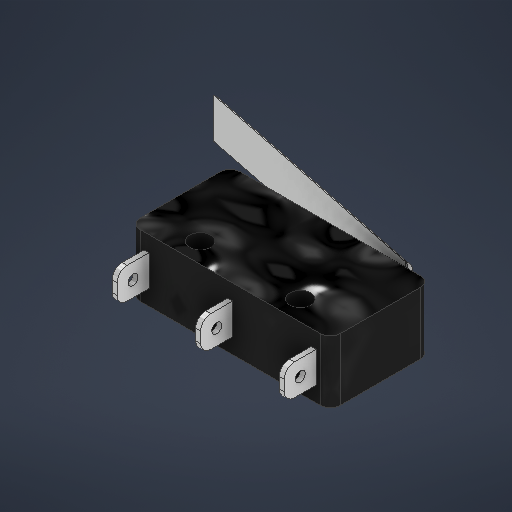
# Autodesk Inventor part: switch
Saved by Autodesk Inventor 2026.1 (Build 301233000, 233)
## iProperties
Created: 2025-11-05
Part Number: switch
Material: Generic
Document SubType Name: Modeling
Designer: Mikke
Density: 1 g/cm^3
Appearance: Default
Author: Mikke
Autodesk Inventor part; units mm, degrees
ref_plane "YZ Plane" through (0, 0, 0) normal (1, 0, 0) x (0, 1, 0)
ref_plane "XZ Plane" through (0, 0, 0) normal (0, 1, 0) x (-1, 0, 0)
ref_plane "XY Plane" through (0, 0, 0) normal (0, 0, 1) x (1, 0, 0)
sketch "Sketch1" plane through (0, 0, 0) normal (0, 1, 0) x (-1, 0, 0)
  line L0 (-10, 5) -> (10, 5)
  line L1 (10, 5) -> (10, -5)
  line L2 (10, -5) -> (-10, -5)
  line L3 (-10, -5) -> (-10, 5)
  line L4 (-10, 5) -> (10, -5) construction
  line L5 (10, 5) -> (-10, -5) construction
  line L6 (10, 5) -> (10, 3)
  line L7 (10, 3) -> (-10, 3)
  line L8 (10, 3) -> (5, 3)
  line L9 (-10, 3) -> (-5, 3)
  circle A0 centre (5, 3) radius 1.05
  circle A1 centre (-5, 3) radius 1.05
  point P0 (0, 0)
  dimension "d0" = 20
  dimension "d1" = 10
  dimension "d2" = 2
  dimension "d3" = 5
  dimension "d4" = 5
  dimension "d5" = 2.1
  dimension "d6" = 2.1
  constraints: 20 end point, 4 point on line, 2 centre point, 2 coincident, 2 midpoint, 2 parallel, 2 perpendicular, 1 horizontal
  measures "d0" distance of L1.end L2.end
  measures "d1" distance of L0.end L1.end
  measures "d2" distance of L0.end L6.end
  measures "d3" distance of L6.end L8.end
  measures "d4" distance of L7.end L9.end
  measures "d5" diameter of A0
  measures "d6" diameter of A1
extrude "Extrusion1" add sketch "Sketch1" along normal blind 6.2 contours L0 L1 L7 A0 A1 L3 | L7 A1 A0 L1 L2 L3
sketch "Sketch2" plane through (-10, 0, 5) normal (0, 0, 1) x (1, 0, 0)
  line L0 (1.65, 1.55) -> (18.35, 1.55)
  line L1 (18.35, 1.55) -> (18.35, 4.65)
  line L2 (18.35, 4.65) -> (1.65, 4.65)
  line L3 (1.65, 4.65) -> (1.65, 1.55)
  line L4 (1.65, 1.55) -> (18.35, 4.65) construction
  line L5 (18.35, 1.55) -> (1.65, 4.65) construction
  line L6 (10.25, 1.55) -> (9.75, 1.55)
  line L7 (9.75, 1.55) -> (9.75, 4.65)
  line L8 (9.75, 4.65) -> (10.25, 4.65)
  line L9 (10.25, 4.65) -> (10.25, 1.55)
  line L10 (10.25, 1.55) -> (9.75, 4.65) construction
  line L11 (9.75, 1.55) -> (10.25, 4.65) construction
  line L12 (1.65, 3.1) -> (18.35, 3.1)
  line L13 (18.1, 1.55) -> (18.6, 1.55)
  line L14 (18.6, 1.55) -> (18.6, 4.65)
  line L15 (18.6, 4.65) -> (18.1, 4.65)
  line L16 (18.1, 4.65) -> (18.1, 1.55)
  line L17 (18.1, 1.55) -> (18.6, 4.65) construction
  line L18 (18.6, 1.55) -> (18.1, 4.65) construction
  line L19 (1.9, 1.55) -> (1.4, 1.55)
  line L20 (1.4, 1.55) -> (1.4, 4.65)
  line L21 (1.4, 4.65) -> (1.9, 4.65)
  line L22 (1.9, 4.65) -> (1.9, 1.55)
  line L23 (1.9, 1.55) -> (1.4, 4.65) construction
  line L24 (1.4, 1.55) -> (1.9, 4.65) construction
  point P0 (10, 0)
  point P1 (10, 3.1)
  point P2 (18.1, 4.6036)
  point P3 (1.9, 1.55)
  point P4 (1.9, 4.65)
  dimension "d9" = 16.7
  dimension "d13" = 0.5
  dimension "d16" = 0.5
  dimension "d17" = 0.5
  constraints: 50 end point, 11 midpoint, 8 parallel, 5 perpendicular, 4 horizontal, 3 point on line
  measures "d9" distance of L2.end L1.end
  measures "d13" distance of L7.end L8.end
  measures "d16" distance of L15.end L14.end
  measures "d17" distance of L20.end L21.end
extrude "Extrusion2" add sketch "Sketch2" along normal blind 3.2 contours L3 L12 L22 L0 | L19 L20 L21 L3 | L3 L2 L22 L12 | L7 L12 L9 L0 | L7 L2 L9 L12 | L16 L12 L1 L0 | L1 L15 L14 L13 | L16 L2 L1 L12
sketch "Sketch4" plane through (8.6, 1.55, 5) normal (1, 0, 0) x (0, 0, -1)
  line L0 (0, 3.1) -> (-3.2, 3.1) projected
  line L1 (0, 0) -> (-3.2, 0) projected
  line L2 (-3.2, 3.1) -> (0, 3.1)
  line L3 (0, 3.1) -> (0, 0)
  line L4 (0, 0) -> (-3.2, 0)
  line L5 (-3.2, 0) -> (-3.2, 3.1)
  circle A0 centre (-1.6, 1.55) radius 0.5
  point P0 (5, -1.55)
  dimension "d18" = 1
  constraints: 8 end point, 2 parallel, 1 centre point, 1 horizontal, 1 perpendicular
  measures "d18" diameter of A0
extrude "Extrusion3" cut sketch "Sketch4" against normal blind 18 contours A0
fillet "Fillet1" radius 1 6 edges at (-8.35, 4.65, 8.2) (-8.35, 1.55, 8.2) (0, 4.65, 8.2) (0, 1.55, 8.2) (8.35, 4.65, 8.2) (8.35, 1.55, 8.2)
sketch "Sketch5" plane through (10, 0, -5) normal (0, 0, -1) x (-1, 0, 0)
  line L0 (0, 6.2) -> (20, 6.2) projected
  line L1 (0, 6.2) -> (3, 6.2)
  line L2 (3, 6.2) -> (3, 0)
  line L3 (0, 0) -> (20, 0) projected
  line L4 (2.75, 1.1) -> (3.25, 1.1)
  line L5 (3.25, 1.1) -> (3.25, 5.1)
  line L6 (3.25, 5.1) -> (2.75, 5.1)
  line L7 (2.75, 5.1) -> (2.75, 1.1)
  line L8 (2.75, 1.1) -> (3.25, 5.1) construction
  line L9 (3.25, 1.1) -> (2.75, 5.1) construction
  point P0 (10, 0)
  point P1 (3, 3.1)
  dimension "d23" = 3
  dimension "d24" = 0.5
  dimension "d25" = 4
  constraints: 16 end point, 3 midpoint, 2 parallel, 2 perpendicular, 2 point on line, 1 horizontal
  measures "d23" distance of L0.start L1.end
  measures "d24" distance of L6.end L5.end
  measures "d25" distance of L5.end L4.end
extrude "Extrusion4" add sketch "Sketch5" along normal blind 1.4
sketch "Sketch6" plane through (10, 0, -6.4) normal (0, 0, -1) x (-1, 0, 0)
  line L0 (2.75, 5.1) -> (3.25, 5.1) projected
  line L1 (3.25, 5.1) -> (3.25, 1.1) projected
  line L2 (2.75, 5.1) -> (3.25, 5.1)
  line L3 (3.25, 5.1) -> (3.25, 1.1)
  line L4 (3.25, 1.1) -> (2.75, 1.1)
  line L5 (2.75, 1.1) -> (2.75, 5.1)
  point P0 (10, 0)
  constraints: 8 end point, 2 parallel, 1 horizontal, 1 perpendicular
sketch "Sketch8" plane through (0, 0, 0) normal (0, 1, 0) x (-1, 0, 0)
  line L0 (-7.25, -6.4) -> (-6.75, -6.4) projected
  line L1 (-7.25, -6.4) -> (17.8, -6.4)
  line L2 (17.8, -6.4) -> (17.8, -11.4)
  line L3 (17.8, -11.4) -> (-7.25, -11.4)
  line L4 (-7.25, -11.4) -> (-7.25, -6.4)
  line L5 (-7.25, -6.4) -> (-6.75, -6.4)
  line L6 (-7, -6.4) -> (17.8, -11.4)
  point P0 (0, 0)
  dimension "d31" = 25.05
  dimension "d32" = 5
  constraints: 12 end point, 3 equal length, 1 horizontal, 1 midpoint, 1 perpendicular
  measures "d31" distance of L2.end L3.end
  measures "d32" distance of L1.end L2.end
sweep "Sweep1" add profiles "Sketch6" path "Sketch8" path curves L6
fillet "Fillet3" radius 1 4 edges at (10, 3.1, -5) (10, 3.1, 5) (-10, 3.1, -5) (-10, 3.1, 5)
fillet "Fillet4" radius 1 2 edges at (7.25, 3.1, -6.4) (6.75, 3.1, -6.4)
body "Solid1"
